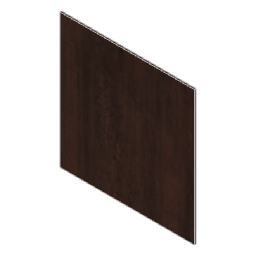
_Plank Barrier 10x10.aca592a7-7670-4089-a1b4-f6026fa7cf75 (Autodesk Fusion 360 design; units mm, degrees)
Autodesk Fusion 360 part; units mm, degrees
sketch "Sketch1" plane through (0, 0, 0) normal (0, 0, 1) x (1, 0, 0)
  line L0 (0, 0) -> (-254, 0)
  line L1 (-254, 0) -> (-254, 3.175)
  line L2 (-254, 3.175) -> (0, 3.175)
  line L3 (0, 3.175) -> (0, 0)
  dimension "d1" = 254
  dimension "d2" = 3.175
  constraint horizontal L0
  constraint vertical L1
  constraint horizontal L2
  constraint vertical L3
  constraint coincident L0.start L3.end
  measures "d1" distance of L0.start L0.end
  measures "d2" distance of L0.start L2.end
extrude "Extrude1" add sketch "Sketch1" along normal blind 254
